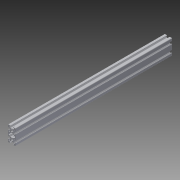
# Autodesk Inventor part: Bosch 20x40 15.5in
Saved by Autodesk Inventor 2015 (Build 190159000, 159)
## iProperties
Created: 2012-09-30
Part Number: Bosch 20x40 15.5in
Material: Aluminum 6061
Document SubType Name: Modeling
Designer: Nemo
Density: 1 g/cm^3
Appearance: Aluminum - Flat
Author: Nemo
Autodesk Inventor part; units mm, degrees
ref_plane "YZ Plane" through (0, 0, 0) normal (1, 0, 0) x (0, 1, 0)
ref_plane "XZ Plane" through (0, 0, 0) normal (0, 1, 0) x (-1, 0, 0)
ref_plane "XY Plane" through (0, 0, 0) normal (0, 0, 1) x (1, 0, 0)
sketch "Bosch 20x40 profile" plane through (0, 0, 0) normal (0, 0, 1) x (1, 0, 0)
  arc A0 (17.5, 27) -> (17, 26.5) centre (17.5, 26.5) ccw
  line L0 (17.8, 27) -> (17.5, 27)
  line L1 (18, 26.7) -> (18, 26.8)
  line L2 (18.3, 26.5) -> (18.2, 26.5)
  arc A1 (18, 26.8) -> (17.8, 27) centre (17.8, 26.8) ccw
  arc A2 (18, 26.7) -> (18.2, 26.5) centre (18.2, 26.7) ccw
  arc A3 (18.5, 26.3) -> (18.3, 26.5) centre (18.3, 26.3) ccw
  arc A4 (12.0858, 25.3535) -> (11.7322, 25.5) centre (11.7322, 25) ccw
  line L3 (11.7322, 25.5) -> (9.4536, 25.5)
  arc A5 (9.7582, 32.4453) -> (7.2418, 32.4453) centre (8.5, 30) ccw
  arc A6 (7.2418, 27.5547) -> (9.7582, 27.5547) centre (8.5, 30) ccw
  arc A7 (17, 35.5) -> (16.5, 36) centre (16.5, 35.5) ccw
  line L4 (15.7678, 36) -> (16.5, 36)
  arc A8 (15.7678, 36) -> (15.4142, 35.8536) centre (15.7678, 35.5) ccw
  line L5 (14.3536, 36.9142) -> (12.0859, 34.6465)
  line L6 (13.1464, 33.5858) -> (15.4142, 35.8536)
  arc A9 (13.1464, 33.5858) -> (13, 33.2322) centre (13.5, 33.2322) ccw
  arc A10 (11.7323, 34.5) -> (12.0859, 34.6465) centre (11.7323, 35) ccw
  arc A11 (2.5, 37.2678) -> (2.6464, 36.9142) centre (3, 37.2678) ccw
  line L7 (2.5, 37.2678) -> (2.5, 38)
  arc A12 (3, 38.5) -> (2.5, 38) centre (3, 38) ccw
  line L8 (3, 38.5) -> (5, 38.5)
  line L9 (4.8, 40) -> (0, 40)
  arc A13 (5, 38.5) -> (5.5, 39) centre (5, 39) ccw
  line L10 (5.5, 39) -> (5.5, 39.3)
  line L11 (5.3, 39.5) -> (5.2, 39.5)
  arc A14 (5.5, 39.3) -> (5.3, 39.5) centre (5.3, 39.3) ccw
  line L12 (5, 39.7) -> (5, 39.8)
  arc A15 (5, 39.7) -> (5.2, 39.5) centre (5.2, 39.7) ccw
  arc A16 (5, 39.8) -> (4.8, 40) centre (4.8, 39.8) ccw
  line L13 (4.9141, 34.6465) -> (2.6464, 36.9142)
  arc A17 (4.9141, 34.6465) -> (5.2677, 34.5) centre (5.2677, 35) ccw
  arc A18 (1.5358, 35.9036) -> (1.1822, 36.05) centre (1.1822, 35.55) ccw
  arc A19 (4, 33.2322) -> (3.8536, 33.5858) centre (3.5, 33.2322) ccw
  line L14 (1.5358, 35.9036) -> (3.8536, 33.5858)
  line L15 (0.5, 36.05) -> (1.1822, 36.05)
  line L16 (5.5523, 31.8871) -> (6.0547, 31.2582)
  arc A20 (6.6129, 32.9477) -> (5.5523, 31.8871) centre (8.5, 30) ccw
  line L17 (7.2418, 32.4453) -> (6.6129, 32.9477)
  line L18 (7.5463, 34.5) -> (5.2677, 34.5)
  arc A21 (7.6463, 34.4733) -> (7.5463, 34.5) centre (7.5463, 34.3) ccw
  arc A22 (8.4, 34.0381) -> (8.6, 34.0381) centre (8.5, 34.2113) ccw
  line L19 (8.4, 34.0381) -> (7.6463, 34.4733)
  line L20 (9.3537, 34.4733) -> (8.6, 34.0381)
  arc A23 (9.4537, 34.5) -> (9.3537, 34.4733) centre (9.4537, 34.3) ccw
  line L21 (4, 33.2322) -> (4, 30.9536)
  line L22 (0, 24.55) -> (0, 26.5)
  arc A24 (0, 24.55) -> (0.5, 24.05) centre (0.5, 24.55) ccw
  line L23 (1.2822, 24.05) -> (0.5, 24.05)
  arc A25 (1.2822, 24.05) -> (1.6358, 24.1964) centre (1.2822, 24.55) ccw
  line L24 (1.8536, 22.5) -> (0.5, 22.5)
  arc A26 (3.8536, 26.4142) -> (4, 26.7678) centre (3.5, 26.7678) ccw
  arc A27 (1.8536, 22.5) -> (2.2071, 22.6464) centre (1.8536, 23) ccw
  line L25 (3.8536, 26.4142) -> (1.6358, 24.1964)
  line L26 (4.9142, 25.3535) -> (2.2071, 22.6464)
  arc A28 (5.2678, 25.5) -> (4.9142, 25.3535) centre (5.2678, 25) ccw
  line L27 (17, 26.5) -> (17, 24.5)
  arc A29 (16.5, 24) -> (17, 24.5) centre (16.5, 24.5) ccw
  line L28 (16.5, 24) -> (15.7678, 24)
  arc A30 (15.4142, 24.1464) -> (15.7678, 24) centre (15.7678, 24.5) ccw
  arc A31 (17, 22) -> (16.5, 22.5) centre (16.5, 22) ccw
  line L29 (16.5, 22.5) -> (15.1464, 22.5)
  line L30 (15.4142, 24.1464) -> (13.1464, 26.4142)
  arc A32 (14.7929, 22.6464) -> (15.1464, 22.5) centre (15.1464, 23) ccw
  line L31 (14.7929, 22.6464) -> (12.0858, 25.3535)
  arc A33 (0, 26.5) -> (-0.5, 27) centre (-0.5, 26.5) ccw
  line L32 (-0.5, 27) -> (-0.8, 27)
  line L33 (-1, 26.8) -> (-1, 26.7)
  arc A34 (-0.8, 27) -> (-1, 26.8) centre (-0.8, 26.8) ccw
  arc A35 (-1.2, 26.5) -> (-1, 26.7) centre (-1.2, 26.7) ccw
  line L34 (-1.2, 26.5) -> (-1.3, 26.5)
  arc A36 (-1.3, 26.5) -> (-1.5, 26.3) centre (-1.3, 26.3) ccw
  line L35 (7.5464, 25.5) -> (5.2678, 25.5)
  line L36 (8.4, 25.9619) -> (7.6464, 25.5268)
  arc A37 (7.5464, 25.5) -> (7.6464, 25.5268) centre (7.5464, 25.7) ccw
  line L37 (9.3536, 25.5268) -> (8.6, 25.9619)
  arc A38 (9.3536, 25.5268) -> (9.4536, 25.5) centre (9.4536, 25.7) ccw
  arc A39 (8.6, 25.9619) -> (8.4, 25.9619) centre (8.5, 25.7887) ccw
  line L38 (11.4477, 28.1129) -> (10.9453, 28.7418)
  line L39 (9.7582, 27.5547) -> (10.3871, 27.0523)
  arc A40 (10.3871, 27.0523) -> (11.4477, 28.1129) centre (8.5, 30) ccw
  arc A41 (13, 26.7678) -> (13.1464, 26.4142) centre (13.5, 26.7678) ccw
  line L40 (13, 26.7678) -> (13, 29.0464)
  arc A42 (10.9453, 28.7418) -> (10.9453, 31.2582) centre (8.5, 30) ccw
  arc A43 (13, 29.0464) -> (12.9732, 29.1464) centre (12.8, 29.0464) ccw
  line L41 (12.9732, 29.1464) -> (12.5381, 29.9)
  arc A44 (12.5381, 30.1) -> (12.5381, 29.9) centre (12.7113, 30) ccw
  line L42 (10.3871, 32.9477) -> (9.7582, 32.4453)
  line L43 (10.9453, 31.2582) -> (11.4477, 31.8871)
  line L44 (12.5381, 30.1) -> (12.9732, 30.8536)
  arc A45 (11.4477, 31.8871) -> (10.3871, 32.9477) centre (8.5, 30) ccw
  arc A46 (12.9732, 30.8536) -> (13, 30.9536) centre (12.8, 30.9536) ccw
  line L45 (13, 30.9536) -> (13, 33.2322)
  arc A47 (4, 30.9536) -> (4.0268, 30.8536) centre (4.2, 30.9536) ccw
  line L46 (4.0268, 30.8536) -> (4.4619, 30.1)
  arc A48 (4.4619, 29.9) -> (4.4619, 30.1) centre (4.2887, 30) ccw
  arc A49 (6.0547, 31.2582) -> (6.0547, 28.7418) centre (8.5, 30) ccw
  line L47 (4.4619, 29.9) -> (4.0268, 29.1464)
  arc A50 (4.0268, 29.1464) -> (4, 29.0464) centre (4.2, 29.0464) ccw
  line L48 (6.0547, 28.7418) -> (5.5523, 28.1129)
  line L49 (6.6129, 27.0523) -> (7.2418, 27.5547)
  arc A51 (5.5523, 28.1129) -> (6.6129, 27.0523) centre (8.5, 30) ccw
  line L50 (4, 29.0464) -> (4, 26.7678)
  arc A52 (0, 40) -> (-1.5, 38.5) centre (0, 38.5) ccw
  line L51 (0, 33.5) -> (0, 35.55)
  arc A53 (-0.5, 33) -> (0, 33.5) centre (-0.5, 33.5) ccw
  line L52 (-0.8, 33) -> (-0.5, 33)
  line L53 (-1, 33.3) -> (-1, 33.2)
  arc A54 (-1, 33.2) -> (-0.8, 33) centre (-0.8, 33.2) ccw
  arc A55 (-1, 33.3) -> (-1.2, 33.5) centre (-1.2, 33.3) ccw
  line L54 (-1.3, 33.5) -> (-1.2, 33.5)
  arc A56 (-1.5, 33.7) -> (-1.3, 33.5) centre (-1.3, 33.7) ccw
  line L55 (-1.5, 38.5) -> (-1.5, 33.7)
  arc A57 (0.5, 36.05) -> (0, 35.55) centre (0.5, 35.55) ccw
  line L56 (11.8, 39.5) -> (11.7, 39.5)
  arc A58 (11.5, 39) -> (12, 38.5) centre (12, 39) ccw
  line L57 (11.5, 39.3) -> (11.5, 39)
  line L58 (11.7323, 34.5) -> (9.4537, 34.5)
  arc A59 (11.7, 39.5) -> (11.5, 39.3) centre (11.7, 39.3) ccw
  line L59 (18.5, 33.7) -> (18.5, 38.5)
  line L60 (17, 35.5) -> (17, 33.5)
  arc A60 (17, 33.5) -> (17.5, 33) centre (17.5, 33.5) ccw
  line L61 (18.2, 33.5) -> (18.3, 33.5)
  line L62 (18, 33.2) -> (18, 33.3)
  line L63 (17.5, 33) -> (17.8, 33)
  arc A61 (18.2, 33.5) -> (18, 33.3) centre (18.2, 33.3) ccw
  arc A62 (18.3, 33.5) -> (18.5, 33.7) centre (18.3, 33.7) ccw
  arc A63 (17.8, 33) -> (18, 33.2) centre (17.8, 33.2) ccw
  arc A64 (18.5, 38.5) -> (17, 40) centre (17, 38.5) ccw
  arc A65 (14.3536, 36.9142) -> (14.5, 37.2678) centre (14, 37.2678) ccw
  line L64 (14.5, 38) -> (14.5, 37.2678)
  line L65 (12, 38.5) -> (14, 38.5)
  arc A66 (14.5, 38) -> (14, 38.5) centre (14, 38) ccw
  arc A67 (11.8, 39.5) -> (12, 39.7) centre (11.8, 39.7) ccw
  line L66 (12, 39.8) -> (12, 39.7)
  arc A68 (12.2, 40) -> (12, 39.8) centre (12.2, 39.8) ccw
  line L67 (17, 40) -> (12.2, 40)
  arc A69 (17, 15.5) -> (16.5, 16) centre (16.5, 15.5) ccw
  arc A70 (15.7678, 16) -> (15.4142, 15.8536) centre (15.7678, 15.5) ccw
  arc A71 (13.1464, 13.5858) -> (13, 13.2322) centre (13.5, 13.2322) ccw
  arc A72 (16.5, 17.5) -> (17, 18) centre (16.5, 18) ccw
  line L68 (15.1464, 17.5) -> (16.5, 17.5)
  line L69 (13.1464, 13.5858) -> (15.4142, 15.8536)
  line L70 (12.086, 14.6466) -> (14.7929, 17.3535)
  arc A73 (15.1464, 17.5) -> (14.7929, 17.3535) centre (15.1464, 17) ccw
  line L71 (18.5, 13.65) -> (18.5, 26.3)
  line L72 (17, 18) -> (17, 22)
  line L73 (15.7678, 16) -> (16.5, 16)
  arc A74 (0.5, 22.5) -> (0, 22) centre (0.5, 22) ccw
  line L74 (-1.5, 26.3) -> (-1.5, 13.65)
  line L75 (0, 22) -> (0, 18)
  line L76 (0, 13.45) -> (0, 15.5)
  arc A75 (0.5, 16) -> (0, 15.5) centre (0.5, 15.5) ccw
  line L77 (0.5, 16) -> (1.2322, 16)
  arc A76 (1.5858, 15.8536) -> (1.2322, 16) centre (1.2322, 15.5) ccw
  arc A77 (0, 18) -> (0.5, 17.5) centre (0.5, 18) ccw
  line L78 (0.5, 17.5) -> (1.8536, 17.5)
  line L79 (1.5858, 15.8536) -> (3.8536, 13.5858)
  arc A78 (2.2071, 17.3535) -> (1.8536, 17.5) centre (1.8536, 17) ccw
  arc A79 (4.914, 14.6466) -> (5.2676, 14.5001) centre (5.2676, 15.0001) ccw
  line L80 (2.2071, 17.3535) -> (4.914, 14.6466)
  line L81 (17, 15.5) -> (17, 13.45)
  line L82 (18.2, 13.45) -> (18.3, 13.45)
  arc A80 (18.3, 13.45) -> (18.5, 13.65) centre (18.3, 13.65) ccw
  arc A81 (18.2, 13.45) -> (18, 13.25) centre (18.2, 13.25) ccw
  line L83 (18, 13.15) -> (18, 13.25)
  arc A82 (17, 13.45) -> (17.5, 12.95) centre (17.5, 13.45) ccw
  line L84 (17.5, 12.95) -> (17.8, 12.95)
  arc A83 (17.8, 12.95) -> (18, 13.15) centre (17.8, 13.15) ccw
  arc A84 (-0.5, 12.95) -> (0, 13.45) centre (-0.5, 13.45) ccw
  line L85 (-1, 13.25) -> (-1, 13.15)
  line L86 (-1.3, 13.45) -> (-1.2, 13.45)
  arc A85 (-1, 13.25) -> (-1.2, 13.45) centre (-1.2, 13.25) ccw
  arc A86 (-1, 13.15) -> (-0.8, 12.95) centre (-0.8, 13.15) ccw
  arc A87 (-1.5, 13.65) -> (-1.3, 13.45) centre (-1.3, 13.65) ccw
  line L87 (-0.8, 12.95) -> (-0.5, 12.95)
  arc A88 (13, 9.0464) -> (12.9732, 9.1464) centre (12.8, 9.0464) ccw
  line L88 (12.9732, 9.1464) -> (12.5381, 9.9)
  arc A89 (12.5381, 10.1) -> (12.5381, 9.9) centre (12.7113, 10) ccw
  line L89 (12.5381, 10.1) -> (12.9732, 10.8536)
  arc A90 (12.9732, 10.8536) -> (13, 10.9536) centre (12.8, 10.9536) ccw
  line L90 (13, 10.9536) -> (13, 13.2322)
  line L91 (9.4538, 14.5001) -> (11.7324, 14.5001)
  arc A91 (11.7324, 14.5001) -> (12.086, 14.6466) centre (11.7324, 15.0001) ccw
  line L92 (7.2418, 12.4453) -> (6.6129, 12.9477)
  line L93 (5.5523, 11.8871) -> (6.0547, 11.2582)
  arc A92 (6.6129, 12.9477) -> (5.5523, 11.8871) centre (8.5, 10) ccw
  line L94 (4, 13.2322) -> (4, 10.9536)
  arc A93 (4, 13.2322) -> (3.8536, 13.5858) centre (3.5, 13.2322) ccw
  arc A94 (6.0547, 11.2582) -> (6.0547, 8.7418) centre (8.5, 10) ccw
  line L95 (6.0547, 8.7418) -> (5.5523, 8.1129)
  arc A95 (5.5523, 8.1129) -> (6.6129, 7.0523) centre (8.5, 10) ccw
  line L96 (6.6129, 7.0523) -> (7.2418, 7.5547)
  arc A96 (9.7582, 12.4453) -> (7.2418, 12.4453) centre (8.5, 10) ccw
  line L97 (10.3871, 12.9477) -> (9.7582, 12.4453)
  arc A97 (11.4477, 11.8871) -> (10.3871, 12.9477) centre (8.5, 10) ccw
  line L98 (10.9453, 11.2582) -> (11.4477, 11.8871)
  arc A98 (10.9453, 8.7418) -> (10.9453, 11.2582) centre (8.5, 10) ccw
  arc A99 (7.2418, 7.5547) -> (9.7582, 7.5547) centre (8.5, 10) ccw
  line L99 (9.7582, 7.5547) -> (10.3871, 7.0523)
  line L100 (11.4477, 8.1129) -> (10.9453, 8.7418)
  arc A100 (10.3871, 7.0523) -> (11.4477, 8.1129) centre (8.5, 10) ccw
  line L101 (13, 6.7678) -> (13, 9.0464)
  line L102 (18, 6.65) -> (18, 6.75)
  arc A101 (17.5, 6.95) -> (17, 6.45) centre (17.5, 6.45) ccw
  line L103 (17.8, 6.95) -> (17.5, 6.95)
  arc A102 (18, 6.75) -> (17.8, 6.95) centre (17.8, 6.75) ccw
  line L104 (18.3, 6.45) -> (18.2, 6.45)
  arc A103 (18, 6.65) -> (18.2, 6.45) centre (18.2, 6.65) ccw
  arc A104 (18.5, 6.25) -> (18.3, 6.45) centre (18.3, 6.25) ccw
  line L105 (4, 9.0464) -> (4, 6.7678)
  arc A105 (4.4619, 9.9) -> (4.4619, 10.1) centre (4.2887, 10) ccw
  line L106 (4.4619, 9.9) -> (4.0268, 9.1464)
  arc A106 (4.0268, 9.1464) -> (4, 9.0464) centre (4.2, 9.0464) ccw
  line L107 (4.0268, 10.8536) -> (4.4619, 10.1)
  arc A107 (4, 10.9536) -> (4.0268, 10.8536) centre (4.2, 10.9536) ccw
  line L108 (5.2678, 5.5) -> (7.5464, 5.5)
  arc A108 (7.5464, 5.5) -> (7.6464, 5.5268) centre (7.5464, 5.7) ccw
  line L109 (7.6464, 5.5268) -> (8.4, 5.9619)
  arc A109 (8.6, 5.9619) -> (8.4, 5.9619) centre (8.5, 5.7887) ccw
  arc A110 (9.3536, 5.5268) -> (9.4536, 5.5) centre (9.4536, 5.7) ccw
  line L110 (9.4536, 5.5) -> (11.7322, 5.5)
  line L111 (8.6, 5.9619) -> (9.3536, 5.5268)
  line L112 (16.5, 4) -> (15.7678, 4)
  arc A111 (15.4142, 4.1464) -> (15.7678, 4) centre (15.7678, 4.5) ccw
  line L113 (12.0858, 5.3536) -> (14.3536, 3.0858)
  arc A112 (12.0858, 5.3536) -> (11.7322, 5.5) centre (11.7322, 5) ccw
  arc A113 (16.5, 4) -> (17, 4.5) centre (16.5, 4.5) ccw
  line L114 (17, 6.45) -> (17, 4.5)
  line L115 (15.4142, 4.1464) -> (13.1464, 6.4142)
  arc A114 (13, 6.7678) -> (13.1464, 6.4142) centre (13.5, 6.7678) ccw
  line L116 (18.5, 1.5) -> (18.5, 6.25)
  arc A115 (14.5, 2.7322) -> (14.3536, 3.0858) centre (14, 2.7322) ccw
  line L117 (14.5, 2.7322) -> (14.5, 2)
  arc A116 (14, 1.5) -> (14.5, 2) centre (14, 2) ccw
  arc A117 (17, 0) -> (18.5, 1.5) centre (17, 1.5) ccw
  line L118 (12.2, 0) -> (17, 0)
  line L119 (14, 1.5) -> (12, 1.5)
  arc A118 (0, 6.45) -> (-0.5, 6.95) centre (-0.5, 6.45) ccw
  line L120 (-0.5, 6.95) -> (-0.8, 6.95)
  line L121 (-1, 6.75) -> (-1, 6.65)
  line L122 (-1.2, 6.45) -> (-1.3, 6.45)
  arc A119 (-1.3, 6.45) -> (-1.5, 6.25) centre (-1.3, 6.25) ccw
  arc A120 (-0.8, 6.95) -> (-1, 6.75) centre (-0.8, 6.75) ccw
  arc A121 (-1.2, 6.45) -> (-1, 6.65) centre (-1.2, 6.65) ccw
  line L123 (12, 0.3) -> (12, 0.2)
  line L124 (11.7, 0.5) -> (11.8, 0.5)
  line L125 (11.5, 1) -> (11.5, 0.7)
  arc A122 (12, 0.3) -> (11.8, 0.5) centre (11.8, 0.3) ccw
  arc A123 (12, 0.2) -> (12.2, 0) centre (12.2, 0.2) ccw
  arc A124 (11.5, 0.7) -> (11.7, 0.5) centre (11.7, 0.7) ccw
  arc A125 (12, 1.5) -> (11.5, 1) centre (12, 1) ccw
  arc A126 (2.6464, 3.0858) -> (2.5, 2.7322) centre (3, 2.7322) ccw
  line L126 (1.2322, 4) -> (0.5, 4)
  arc A127 (1.2322, 4) -> (1.5858, 4.1464) centre (1.2322, 4.5) ccw
  arc A128 (0, 4.5) -> (0.5, 4) centre (0.5, 4.5) ccw
  line L127 (-1.5, 6.25) -> (-1.5, 1.5)
  line L128 (2.6464, 3.0858) -> (4.9142, 5.3536)
  line L129 (0, 4.5) -> (0, 6.45)
  line L130 (3.8536, 6.4142) -> (1.5858, 4.1464)
  arc A129 (3.8536, 6.4142) -> (4, 6.7678) centre (3.5, 6.7678) ccw
  arc A130 (5.2678, 5.5) -> (4.9142, 5.3536) centre (5.2678, 5) ccw
  line L131 (2.5, 2) -> (2.5, 2.7322)
  line L132 (5, 1.5) -> (3, 1.5)
  arc A131 (2.5, 2) -> (3, 1.5) centre (3, 2) ccw
  arc A132 (5.5, 1) -> (5, 1.5) centre (5, 1) ccw
  line L133 (5.5, 0.7) -> (5.5, 1)
  arc A133 (5.3, 0.5) -> (5.5, 0.7) centre (5.3, 0.7) ccw
  line L134 (5.2, 0.5) -> (5.3, 0.5)
  arc A134 (5.2, 0.5) -> (5, 0.3) centre (5.2, 0.3) ccw
  line L135 (5, 0.2) -> (5, 0.3)
  arc A135 (4.8, 0) -> (5, 0.2) centre (4.8, 0.2) ccw
  line L136 (0, 0) -> (4.8, 0)
  arc A136 (-1.5, 1.5) -> (0, 0) centre (0, 1.5) ccw
  arc A137 (9.4538, 14.5001) -> (9.3538, 14.4733) centre (9.4538, 14.3001) ccw
  line L137 (8.6, 14.0381) -> (9.3538, 14.4733)
  arc A138 (8.4, 14.0381) -> (8.6, 14.0381) centre (8.5, 14.2113) ccw
  line L138 (7.6462, 14.4733) -> (8.4, 14.0381)
  arc A139 (7.6462, 14.4733) -> (7.5462, 14.5001) centre (7.5462, 14.3001) ccw
  line L139 (5.2676, 14.5001) -> (7.5462, 14.5001)
  point P0 (8.5, 19.9957)
sketch "Sketch1" plane through (0, 0, 0) normal (0, 0, 1) x (1, 0, 0)
  arc A0 (9, 7.0043) -> (8.5, 6.5043) centre (9, 6.5043) ccw
  line L0 (9.3, 7.0043) -> (9, 7.0043)
  line L1 (9.5, 6.7043) -> (9.5, 6.8043)
  line L2 (9.8, 6.5043) -> (9.7, 6.5043)
  arc A1 (9.5, 6.8043) -> (9.3, 7.0043) centre (9.3, 6.8043) ccw
  arc A2 (9.5, 6.7043) -> (9.7, 6.5043) centre (9.7, 6.7043) ccw
  arc A3 (10, 6.3043) -> (9.8, 6.5043) centre (9.8, 6.3043) ccw
  arc A4 (3.5858, 5.3578) -> (3.2322, 5.5043) centre (3.2322, 5.0043) ccw
  line L3 (3.2322, 5.5043) -> (0.9536, 5.5043)
  arc A5 (1.2582, 12.4496) -> (-1.2582, 12.4496) centre (0, 10.0043) ccw
  arc A6 (-1.2582, 7.559) -> (1.2582, 7.559) centre (0, 10.0043) ccw
  arc A7 (8.5, 15.5043) -> (8, 16.0043) centre (8, 15.5043) ccw
  line L4 (7.2678, 16.0043) -> (8, 16.0043)
  arc A8 (7.2678, 16.0043) -> (6.9142, 15.8578) centre (7.2678, 15.5043) ccw
  line L5 (5.8536, 16.9185) -> (3.5859, 14.6508)
  line L6 (4.6464, 13.5901) -> (6.9142, 15.8578)
  arc A9 (4.6464, 13.5901) -> (4.5, 13.2365) centre (5, 13.2365) ccw
  arc A10 (3.2323, 14.5043) -> (3.5859, 14.6508) centre (3.2323, 15.0043) ccw
  arc A11 (-6, 17.272) -> (-5.8536, 16.9185) centre (-5.5, 17.272) ccw
  line L7 (-6, 17.272) -> (-6, 18.0043)
  arc A12 (-5.5, 18.5043) -> (-6, 18.0043) centre (-5.5, 18.0043) ccw
  line L8 (-5.5, 18.5043) -> (-3.5, 18.5043)
  line L9 (-3.7, 20.0043) -> (-8.5, 20.0043)
  arc A13 (-3.5, 18.5043) -> (-3, 19.0043) centre (-3.5, 19.0043) ccw
  line L10 (-3, 19.0043) -> (-3, 19.3043)
  line L11 (-3.2, 19.5043) -> (-3.3, 19.5043)
  arc A14 (-3, 19.3043) -> (-3.2, 19.5043) centre (-3.2, 19.3043) ccw
  line L12 (-3.5, 19.7043) -> (-3.5, 19.8043)
  arc A15 (-3.5, 19.7043) -> (-3.3, 19.5043) centre (-3.3, 19.7043) ccw
  arc A16 (-3.5, 19.8043) -> (-3.7, 20.0043) centre (-3.7, 19.8043) ccw
  line L13 (-3.5859, 14.6508) -> (-5.8536, 16.9185)
  arc A17 (-3.5859, 14.6508) -> (-3.2323, 14.5043) centre (-3.2323, 15.0043) ccw
  arc A18 (-6.9642, 15.9078) -> (-7.3178, 16.0543) centre (-7.3178, 15.5543) ccw
  arc A19 (-4.5, 13.2365) -> (-4.6464, 13.5901) centre (-5, 13.2365) ccw
  line L14 (-6.9642, 15.9078) -> (-4.6464, 13.5901)
  line L15 (-8, 16.0543) -> (-7.3178, 16.0543)
  line L16 (-2.9477, 11.8913) -> (-2.4453, 11.2625)
  arc A20 (-1.8871, 12.952) -> (-2.9477, 11.8913) centre (0, 10.0043) ccw
  line L17 (-1.2582, 12.4496) -> (-1.8871, 12.952)
  line L18 (-0.9537, 14.5043) -> (-3.2323, 14.5043)
  arc A21 (-0.8537, 14.4775) -> (-0.9537, 14.5043) centre (-0.9537, 14.3043) ccw
  arc A22 (-0.1, 14.0424) -> (0.1, 14.0424) centre (0, 14.2156) ccw
  line L19 (-0.1, 14.0424) -> (-0.8537, 14.4775)
  line L20 (0.8537, 14.4775) -> (0.1, 14.0424)
  arc A23 (0.9537, 14.5043) -> (0.8537, 14.4775) centre (0.9537, 14.3043) ccw
  line L21 (-4.5, 13.2365) -> (-4.5, 10.9579)
  line L22 (-8.5, 4.5543) -> (-8.5, 6.5043)
  arc A24 (-8.5, 4.5543) -> (-8, 4.0543) centre (-8, 4.5543) ccw
  line L23 (-7.2178, 4.0543) -> (-8, 4.0543)
  arc A25 (-7.2178, 4.0543) -> (-6.8642, 4.2007) centre (-7.2178, 4.5543) ccw
  line L24 (-6.6464, 2.5043) -> (-8, 2.5043)
  arc A26 (-4.6464, 6.4185) -> (-4.5, 6.7721) centre (-5, 6.7721) ccw
  arc A27 (-6.6464, 2.5043) -> (-6.2929, 2.6507) centre (-6.6464, 3.0043) ccw
  line L25 (-4.6464, 6.4185) -> (-6.8642, 4.2007)
  line L26 (-3.5858, 5.3578) -> (-6.2929, 2.6507)
  arc A28 (-3.2322, 5.5043) -> (-3.5858, 5.3578) centre (-3.2322, 5.0043) ccw
  line L27 (8.5, 6.5043) -> (8.5, 4.5043)
  arc A29 (8, 4.0043) -> (8.5, 4.5043) centre (8, 4.5043) ccw
  line L28 (8, 4.0043) -> (7.2678, 4.0043)
  arc A30 (6.9142, 4.1507) -> (7.2678, 4.0043) centre (7.2678, 4.5043) ccw
  arc A31 (8.5, 2.0043) -> (8, 2.5043) centre (8, 2.0043) ccw
  line L29 (8, 2.5043) -> (6.6464, 2.5043)
  line L30 (6.9142, 4.1507) -> (4.6464, 6.4185)
  arc A32 (6.2929, 2.6507) -> (6.6464, 2.5043) centre (6.6464, 3.0043) ccw
  line L31 (6.2929, 2.6507) -> (3.5858, 5.3578)
  arc A33 (-8.5, 6.5043) -> (-9, 7.0043) centre (-9, 6.5043) ccw
  line L32 (-9, 7.0043) -> (-9.3, 7.0043)
  line L33 (-9.5, 6.8043) -> (-9.5, 6.7043)
  arc A34 (-9.3, 7.0043) -> (-9.5, 6.8043) centre (-9.3, 6.8043) ccw
  arc A35 (-9.7, 6.5043) -> (-9.5, 6.7043) centre (-9.7, 6.7043) ccw
  line L34 (-9.7, 6.5043) -> (-9.8, 6.5043)
  arc A36 (-9.8, 6.5043) -> (-10, 6.3043) centre (-9.8, 6.3043) ccw
  line L35 (-0.9536, 5.5043) -> (-3.2322, 5.5043)
  line L36 (-0.1, 5.9662) -> (-0.8536, 5.5311)
  arc A37 (-0.9536, 5.5043) -> (-0.8536, 5.5311) centre (-0.9536, 5.7043) ccw
  line L37 (0.8536, 5.5311) -> (0.1, 5.9662)
  arc A38 (0.8536, 5.5311) -> (0.9536, 5.5043) centre (0.9536, 5.7043) ccw
  arc A39 (0.1, 5.9662) -> (-0.1, 5.9662) centre (0, 5.793) ccw
  line L38 (2.9477, 8.1172) -> (2.4453, 8.7461)
  line L39 (1.2582, 7.559) -> (1.8871, 7.0566)
  arc A40 (1.8871, 7.0566) -> (2.9477, 8.1172) centre (0, 10.0043) ccw
  arc A41 (4.5, 6.7721) -> (4.6464, 6.4185) centre (5, 6.7721) ccw
  line L40 (4.5, 6.7721) -> (4.5, 9.0507)
  arc A42 (2.4453, 8.7461) -> (2.4453, 11.2625) centre (0, 10.0043) ccw
  arc A43 (4.5, 9.0507) -> (4.4732, 9.1507) centre (4.3, 9.0507) ccw
  line L41 (4.4732, 9.1507) -> (4.0381, 9.9043)
  arc A44 (4.0381, 10.1043) -> (4.0381, 9.9043) centre (4.2113, 10.0043) ccw
  line L42 (1.8871, 12.952) -> (1.2582, 12.4496)
  line L43 (2.4453, 11.2625) -> (2.9477, 11.8913)
  line L44 (4.0381, 10.1043) -> (4.4732, 10.8579)
  arc A45 (2.9477, 11.8913) -> (1.8871, 12.952) centre (0, 10.0043) ccw
  arc A46 (4.4732, 10.8579) -> (4.5, 10.9579) centre (4.3, 10.9579) ccw
  line L45 (4.5, 10.9579) -> (4.5, 13.2365)
  arc A47 (-4.5, 10.9579) -> (-4.4732, 10.8579) centre (-4.3, 10.9579) ccw
  line L46 (-4.4732, 10.8579) -> (-4.0381, 10.1043)
  arc A48 (-4.0381, 9.9043) -> (-4.0381, 10.1043) centre (-4.2113, 10.0043) ccw
  arc A49 (-2.4453, 11.2625) -> (-2.4453, 8.7461) centre (0, 10.0043) ccw
  line L47 (-4.0381, 9.9043) -> (-4.4732, 9.1507)
  arc A50 (-4.4732, 9.1507) -> (-4.5, 9.0507) centre (-4.3, 9.0507) ccw
  line L48 (-2.4453, 8.7461) -> (-2.9477, 8.1172)
  line L49 (-1.8871, 7.0566) -> (-1.2582, 7.559)
  arc A51 (-2.9477, 8.1172) -> (-1.8871, 7.0566) centre (0, 10.0043) ccw
  line L50 (-4.5, 9.0507) -> (-4.5, 6.7721)
  arc A52 (-8.5, 20.0043) -> (-10, 18.5043) centre (-8.5, 18.5043) ccw
  line L51 (-8.5, 13.5043) -> (-8.5, 15.5543)
  arc A53 (-9, 13.0043) -> (-8.5, 13.5043) centre (-9, 13.5043) ccw
  line L52 (-9.3, 13.0043) -> (-9, 13.0043)
  line L53 (-9.5, 13.3043) -> (-9.5, 13.2043)
  arc A54 (-9.5, 13.2043) -> (-9.3, 13.0043) centre (-9.3, 13.2043) ccw
  arc A55 (-9.5, 13.3043) -> (-9.7, 13.5043) centre (-9.7, 13.3043) ccw
  line L54 (-9.8, 13.5043) -> (-9.7, 13.5043)
  arc A56 (-10, 13.7043) -> (-9.8, 13.5043) centre (-9.8, 13.7043) ccw
  line L55 (-10, 18.5043) -> (-10, 13.7043)
  arc A57 (-8, 16.0543) -> (-8.5, 15.5543) centre (-8, 15.5543) ccw
  line L56 (3.3, 19.5043) -> (3.2, 19.5043)
  arc A58 (3, 19.0043) -> (3.5, 18.5043) centre (3.5, 19.0043) ccw
  line L57 (3, 19.3043) -> (3, 19.0043)
  line L58 (3.2323, 14.5043) -> (0.9537, 14.5043)
  arc A59 (3.2, 19.5043) -> (3, 19.3043) centre (3.2, 19.3043) ccw
  line L59 (10, 13.7043) -> (10, 18.5043)
  line L60 (8.5, 15.5043) -> (8.5, 13.5043)
  arc A60 (8.5, 13.5043) -> (9, 13.0043) centre (9, 13.5043) ccw
  line L61 (9.7, 13.5043) -> (9.8, 13.5043)
  line L62 (9.5, 13.2043) -> (9.5, 13.3043)
  line L63 (9, 13.0043) -> (9.3, 13.0043)
  arc A61 (9.7, 13.5043) -> (9.5, 13.3043) centre (9.7, 13.3043) ccw
  arc A62 (9.8, 13.5043) -> (10, 13.7043) centre (9.8, 13.7043) ccw
  arc A63 (9.3, 13.0043) -> (9.5, 13.2043) centre (9.3, 13.2043) ccw
  arc A64 (10, 18.5043) -> (8.5, 20.0043) centre (8.5, 18.5043) ccw
  arc A65 (5.8536, 16.9185) -> (6, 17.272) centre (5.5, 17.272) ccw
  line L64 (6, 18.0043) -> (6, 17.272)
  line L65 (3.5, 18.5043) -> (5.5, 18.5043)
  arc A66 (6, 18.0043) -> (5.5, 18.5043) centre (5.5, 18.0043) ccw
  arc A67 (3.3, 19.5043) -> (3.5, 19.7043) centre (3.3, 19.7043) ccw
  line L66 (3.5, 19.8043) -> (3.5, 19.7043)
  arc A68 (3.7, 20.0043) -> (3.5, 19.8043) centre (3.7, 19.8043) ccw
  line L67 (8.5, 20.0043) -> (3.7, 20.0043)
  arc A69 (8.5, -4.4957) -> (8, -3.9957) centre (8, -4.4957) ccw
  arc A70 (7.2678, -3.9957) -> (6.9142, -4.1422) centre (7.2678, -4.4957) ccw
  arc A71 (4.6464, -6.4099) -> (4.5, -6.7635) centre (5, -6.7635) ccw
  arc A72 (8, -2.4957) -> (8.5, -1.9957) centre (8, -1.9957) ccw
  line L68 (6.6464, -2.4957) -> (8, -2.4957)
  line L69 (4.6464, -6.4099) -> (6.9142, -4.1422)
  line L70 (3.586, -5.3492) -> (6.2929, -2.6422)
  arc A73 (6.6464, -2.4957) -> (6.2929, -2.6422) centre (6.6464, -2.9957) ccw
  line L71 (10, -6.3457) -> (10, 6.3043)
  line L72 (8.5, -1.9957) -> (8.5, 2.0043)
  line L73 (7.2678, -3.9957) -> (8, -3.9957)
  arc A74 (-8, 2.5043) -> (-8.5, 2.0043) centre (-8, 2.0043) ccw
  line L74 (-10, 6.3043) -> (-10, -6.3457)
  line L75 (-8.5, 2.0043) -> (-8.5, -1.9957)
  line L76 (-8.5, -6.5457) -> (-8.5, -4.4957)
  arc A75 (-8, -3.9957) -> (-8.5, -4.4957) centre (-8, -4.4957) ccw
  line L77 (-8, -3.9957) -> (-7.2678, -3.9957)
  arc A76 (-6.9142, -4.1422) -> (-7.2678, -3.9957) centre (-7.2678, -4.4957) ccw
  arc A77 (-8.5, -1.9957) -> (-8, -2.4957) centre (-8, -1.9957) ccw
  line L78 (-8, -2.4957) -> (-6.6464, -2.4957)
  line L79 (-6.9142, -4.1422) -> (-4.6464, -6.4099)
  arc A78 (-6.2929, -2.6422) -> (-6.6464, -2.4957) centre (-6.6464, -2.9957) ccw
  arc A79 (-3.586, -5.3492) -> (-3.2324, -5.4956) centre (-3.2324, -4.9956) ccw
  line L80 (-6.2929, -2.6422) -> (-3.586, -5.3492)
  line L81 (8.5, -4.4957) -> (8.5, -6.5457)
  line L82 (9.7, -6.5457) -> (9.8, -6.5457)
  arc A80 (9.8, -6.5457) -> (10, -6.3457) centre (9.8, -6.3457) ccw
  arc A81 (9.7, -6.5457) -> (9.5, -6.7457) centre (9.7, -6.7457) ccw
  line L83 (9.5, -6.8457) -> (9.5, -6.7457)
  arc A82 (8.5, -6.5457) -> (9, -7.0457) centre (9, -6.5457) ccw
  line L84 (9, -7.0457) -> (9.3, -7.0457)
  arc A83 (9.3, -7.0457) -> (9.5, -6.8457) centre (9.3, -6.8457) ccw
  arc A84 (-9, -7.0457) -> (-8.5, -6.5457) centre (-9, -6.5457) ccw
  line L85 (-9.5, -6.7457) -> (-9.5, -6.8457)
  line L86 (-9.8, -6.5457) -> (-9.7, -6.5457)
  arc A85 (-9.5, -6.7457) -> (-9.7, -6.5457) centre (-9.7, -6.7457) ccw
  arc A86 (-9.5, -6.8457) -> (-9.3, -7.0457) centre (-9.3, -6.8457) ccw
  arc A87 (-10, -6.3457) -> (-9.8, -6.5457) centre (-9.8, -6.3457) ccw
  line L87 (-9.3, -7.0457) -> (-9, -7.0457)
  arc A88 (4.5, -10.9493) -> (4.4732, -10.8493) centre (4.3, -10.9493) ccw
  line L88 (4.4732, -10.8493) -> (4.0381, -10.0957)
  arc A89 (4.0381, -9.8957) -> (4.0381, -10.0957) centre (4.2113, -9.9957) ccw
  line L89 (4.0381, -9.8957) -> (4.4732, -9.1421)
  arc A90 (4.4732, -9.1421) -> (4.5, -9.0421) centre (4.3, -9.0421) ccw
  line L90 (4.5, -9.0421) -> (4.5, -6.7635)
  line L91 (0.9538, -5.4956) -> (3.2324, -5.4956)
  arc A91 (3.2324, -5.4956) -> (3.586, -5.3492) centre (3.2324, -4.9956) ccw
  line L92 (-1.2582, -7.5504) -> (-1.8871, -7.048)
  line L93 (-2.9477, -8.1087) -> (-2.4453, -8.7375)
  arc A92 (-1.8871, -7.048) -> (-2.9477, -8.1087) centre (0, -9.9957) ccw
  line L94 (-4.5, -6.7635) -> (-4.5, -9.0421)
  arc A93 (-4.5, -6.7635) -> (-4.6464, -6.4099) centre (-5, -6.7635) ccw
  arc A94 (-2.4453, -8.7375) -> (-2.4453, -11.2539) centre (0, -9.9957) ccw
  line L95 (-2.4453, -11.2539) -> (-2.9477, -11.8828)
  arc A95 (-2.9477, -11.8828) -> (-1.8871, -12.9434) centre (0, -9.9957) ccw
  line L96 (-1.8871, -12.9434) -> (-1.2582, -12.441)
  arc A96 (1.2582, -7.5504) -> (-1.2582, -7.5504) centre (0, -9.9957) ccw
  line L97 (1.8871, -7.048) -> (1.2582, -7.5504)
  arc A97 (2.9477, -8.1087) -> (1.8871, -7.048) centre (0, -9.9957) ccw
  line L98 (2.4453, -8.7375) -> (2.9477, -8.1087)
  arc A98 (2.4453, -11.2539) -> (2.4453, -8.7375) centre (0, -9.9957) ccw
  arc A99 (-1.2582, -12.441) -> (1.2582, -12.441) centre (0, -9.9957) ccw
  line L99 (1.2582, -12.441) -> (1.8871, -12.9434)
  line L100 (2.9477, -11.8828) -> (2.4453, -11.2539)
  arc A100 (1.8871, -12.9434) -> (2.9477, -11.8828) centre (0, -9.9957) ccw
  line L101 (4.5, -13.2279) -> (4.5, -10.9493)
  line L102 (9.5, -13.3457) -> (9.5, -13.2457)
  arc A101 (9, -13.0457) -> (8.5, -13.5457) centre (9, -13.5457) ccw
  line L103 (9.3, -13.0457) -> (9, -13.0457)
  arc A102 (9.5, -13.2457) -> (9.3, -13.0457) centre (9.3, -13.2457) ccw
  line L104 (9.8, -13.5457) -> (9.7, -13.5457)
  arc A103 (9.5, -13.3457) -> (9.7, -13.5457) centre (9.7, -13.3457) ccw
  arc A104 (10, -13.7457) -> (9.8, -13.5457) centre (9.8, -13.7457) ccw
  line L105 (-4.5, -10.9493) -> (-4.5, -13.2279)
  arc A105 (-4.0381, -10.0957) -> (-4.0381, -9.8957) centre (-4.2113, -9.9957) ccw
  line L106 (-4.0381, -10.0957) -> (-4.4732, -10.8493)
  arc A106 (-4.4732, -10.8493) -> (-4.5, -10.9493) centre (-4.3, -10.9493) ccw
  line L107 (-4.4732, -9.1421) -> (-4.0381, -9.8957)
  arc A107 (-4.5, -9.0421) -> (-4.4732, -9.1421) centre (-4.3, -9.0421) ccw
  line L108 (-3.2322, -14.4957) -> (-0.9536, -14.4957)
  arc A108 (-0.9536, -14.4957) -> (-0.8536, -14.4689) centre (-0.9536, -14.2957) ccw
  line L109 (-0.8536, -14.4689) -> (-0.1, -14.0338)
  arc A109 (0.1, -14.0338) -> (-0.1, -14.0338) centre (0, -14.207) ccw
  arc A110 (0.8536, -14.4689) -> (0.9536, -14.4957) centre (0.9536, -14.2957) ccw
  line L110 (0.9536, -14.4957) -> (3.2322, -14.4957)
  line L111 (0.1, -14.0338) -> (0.8536, -14.4689)
  line L112 (8, -15.9957) -> (7.2678, -15.9957)
  arc A111 (6.9142, -15.8493) -> (7.2678, -15.9957) centre (7.2678, -15.4957) ccw
  line L113 (3.5858, -14.6422) -> (5.8536, -16.9099)
  arc A112 (3.5858, -14.6422) -> (3.2322, -14.4957) centre (3.2322, -14.9957) ccw
  arc A113 (8, -15.9957) -> (8.5, -15.4957) centre (8, -15.4957) ccw
  line L114 (8.5, -13.5457) -> (8.5, -15.4957)
  line L115 (6.9142, -15.8493) -> (4.6464, -13.5815)
  arc A114 (4.5, -13.2279) -> (4.6464, -13.5815) centre (5, -13.2279) ccw
  line L116 (10, -18.4957) -> (10, -13.7457)
  arc A115 (6, -17.2635) -> (5.8536, -16.9099) centre (5.5, -17.2635) ccw
  line L117 (6, -17.2635) -> (6, -17.9957)
  arc A116 (5.5, -18.4957) -> (6, -17.9957) centre (5.5, -17.9957) ccw
  arc A117 (8.5, -19.9957) -> (10, -18.4957) centre (8.5, -18.4957) ccw
  line L118 (3.7, -19.9957) -> (8.5, -19.9957)
  line L119 (5.5, -18.4957) -> (3.5, -18.4957)
  arc A118 (-8.5, -13.5457) -> (-9, -13.0457) centre (-9, -13.5457) ccw
  line L120 (-9, -13.0457) -> (-9.3, -13.0457)
  line L121 (-9.5, -13.2457) -> (-9.5, -13.3457)
  line L122 (-9.7, -13.5457) -> (-9.8, -13.5457)
  arc A119 (-9.8, -13.5457) -> (-10, -13.7457) centre (-9.8, -13.7457) ccw
  arc A120 (-9.3, -13.0457) -> (-9.5, -13.2457) centre (-9.3, -13.2457) ccw
  arc A121 (-9.7, -13.5457) -> (-9.5, -13.3457) centre (-9.7, -13.3457) ccw
  line L123 (3.5, -19.6957) -> (3.5, -19.7957)
  line L124 (3.2, -19.4957) -> (3.3, -19.4957)
  line L125 (3, -18.9957) -> (3, -19.2957)
  arc A122 (3.5, -19.6957) -> (3.3, -19.4957) centre (3.3, -19.6957) ccw
  arc A123 (3.5, -19.7957) -> (3.7, -19.9957) centre (3.7, -19.7957) ccw
  arc A124 (3, -19.2957) -> (3.2, -19.4957) centre (3.2, -19.2957) ccw
  arc A125 (3.5, -18.4957) -> (3, -18.9957) centre (3.5, -18.9957) ccw
  arc A126 (-5.8536, -16.9099) -> (-6, -17.2635) centre (-5.5, -17.2635) ccw
  line L126 (-7.2678, -15.9957) -> (-8, -15.9957)
  arc A127 (-7.2678, -15.9957) -> (-6.9142, -15.8493) centre (-7.2678, -15.4957) ccw
  arc A128 (-8.5, -15.4957) -> (-8, -15.9957) centre (-8, -15.4957) ccw
  line L127 (-10, -13.7457) -> (-10, -18.4957)
  line L128 (-5.8536, -16.9099) -> (-3.5858, -14.6422)
  line L129 (-8.5, -15.4957) -> (-8.5, -13.5457)
  line L130 (-4.6464, -13.5815) -> (-6.9142, -15.8493)
  arc A129 (-4.6464, -13.5815) -> (-4.5, -13.2279) centre (-5, -13.2279) ccw
  arc A130 (-3.2322, -14.4957) -> (-3.5858, -14.6422) centre (-3.2322, -14.9957) ccw
  line L131 (-6, -17.9957) -> (-6, -17.2635)
  line L132 (-3.5, -18.4957) -> (-5.5, -18.4957)
  arc A131 (-6, -17.9957) -> (-5.5, -18.4957) centre (-5.5, -17.9957) ccw
  arc A132 (-3, -18.9957) -> (-3.5, -18.4957) centre (-3.5, -18.9957) ccw
  line L133 (-3, -19.2957) -> (-3, -18.9957)
  arc A133 (-3.2, -19.4957) -> (-3, -19.2957) centre (-3.2, -19.2957) ccw
  line L134 (-3.3, -19.4957) -> (-3.2, -19.4957)
  arc A134 (-3.3, -19.4957) -> (-3.5, -19.6957) centre (-3.3, -19.6957) ccw
  line L135 (-3.5, -19.7957) -> (-3.5, -19.6957)
  arc A135 (-3.7, -19.9957) -> (-3.5, -19.7957) centre (-3.7, -19.7957) ccw
  line L136 (-8.5, -19.9957) -> (-3.7, -19.9957)
  arc A136 (-10, -18.4957) -> (-8.5, -19.9957) centre (-8.5, -18.4957) ccw
  arc A137 (0.9538, -5.4956) -> (0.8538, -5.5224) centre (0.9538, -5.6956) ccw
  line L137 (0.1, -5.9576) -> (0.8538, -5.5224)
  arc A138 (-0.1, -5.9576) -> (0.1, -5.9576) centre (0, -5.7844) ccw
  line L138 (-0.8538, -5.5224) -> (-0.1, -5.9576)
  arc A139 (-0.8538, -5.5224) -> (-0.9538, -5.4956) centre (-0.9538, -5.6956) ccw
  line L139 (-3.2324, -5.4956) -> (-0.9538, -5.4956)
  point P0 (0, 0)
extrude "Extrusion1" add sketch "Sketch1" along normal mid plane 409.702
sketch "Sketch2" plane through (3.7, 20.0043, 204.851) normal (0, 1, 0) x (1, 0, 0)
  line L0 (-3.6, 0) -> (-3.8, 0) projected
  line L1 (-0.4677, 0) -> (-2.7463, 0) projected
  point P0 (-3.7, 204.851)
  point P1 (-3.7, 8.001)
  point P2 (-3.7, 24.003)
  dimension "d10" = 24.003
  dimension "d11" = 16.002
  measures "d10" distance from line of L1 point (-3.7, 24.003)
  measures "d11" distance of point (-3.7, 8.001) point (-3.7, 24.003)
hole "Hole1" at (0, 20.0043, 196.85) at (0, 20.0043, 180.848) direction (0, -1, 0) diameter 4.3656 end through all
body "Solid1"
